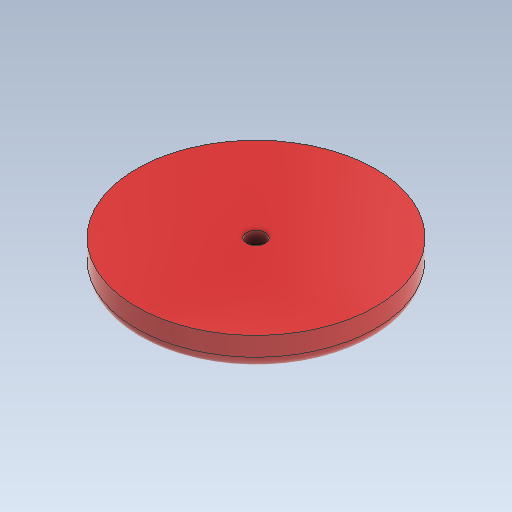
# Autodesk Inventor part: Seal_M_TPU
Saved by Autodesk Inventor 2020 (Build 240168000, 168)
## iProperties
Created: 2020-05-05
Part Number: Seal_M_TPU
Material: Generic
Document SubType Name: Modeling
Designer: Theo Cominotto
Density: 1 g/cm^3
Appearance: Default
Author: Theo Cominotto
Autodesk Inventor part; units mm, degrees
ref_plane "YZ Plane" through (0, 0, 0) normal (1, 0, 0) x (0, 1, 0)
ref_plane "XZ Plane" through (0, 0, 0) normal (0, 1, 0) x (-1, 0, 0)
ref_plane "XY Plane" through (0, 0, 0) normal (0, 0, 1) x (1, 0, 0)
sketch "Sketch1" plane through (0, 0, 0) normal (0, 0, 1) x (1, 0, 0)
  line L0 (0, 0) -> (19, 0)
  line L1 (0, 0) -> (0, -2)
  line L2 (0, -2) -> (13, -2)
  line L3 (13, -2) -> (13, -5)
  line L4 (13, -5) -> (17, -5)
  line L5 (19, -3) -> (19, 0)
  line L6 (1.5, 0) -> (1.5, -2)
  arc A0 (17, -5) -> (19, -3) centre (17, -3) ccw
  point P0 (19, -5)
  dimension "d5" = 19
  dimension "d12" = 2
  dimension "d16" = 5
  dimension "d17" = 1.5
  dimension "d23" = 2
  dimension "d24" = 90
  dimension "d25" = 4
  constraints: 14 end point, 4 point on line, 3 perpendicular, 2 point on circle, 2 tangent, 1 centre point, 1 horizontal, 1 vertical
  measures "d5" distance of L0.start L0.end
  measures "d12" distance of L0.start L1.end
  measures "d16" distance between parallel lines of L0 L4
  measures "d17" distance between parallel lines of L1 L6
  measures "d23" radius of A0
  measures "d24" angle of L3 L2
  measures "d25" distance of L3.end L4.end
revolve "Revolution1" add sketch "Sketch1" angle 360 about axis through (0, 0, 0) along (0, -1, 0) contours L0 L5 A0 L4 L3 L2 L6
fillet "Fillet2" radius 0.5 1 edges at (-13, -5, 0)
fillet "Fillet3" radius 2 1 edges at (-13, -2, 0)
body "Solid1"
